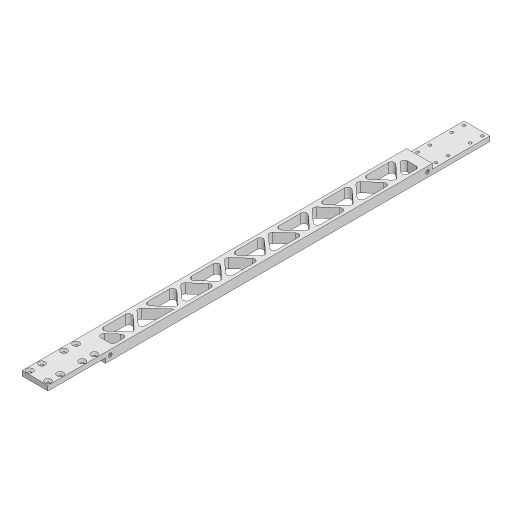
# Autodesk Inventor part: mgn7 300mm Connector Plate
Saved by Autodesk Inventor 2023 (Build 270158000, 158)
## iProperties
Created: 2022-09-25
Part Number: mgn7 300mm Connector Plate
Material: Generic
Document SubType Name: Modeling
Designer: deli
Density: 1 g/cm^3
Appearance: Default
Mass: 15.4529 g
Surface Area: 147.421 cm^2
Volume: 15.4529 cm^3
Author: deli
Autodesk Inventor part; units mm, degrees
ref_plane "YZ Plane" through (0, 0, 0) normal (1, 0, 0) x (0, 1, 0)
ref_plane "XZ Plane" through (0, 0, 0) normal (0, 1, 0) x (-1, 0, 0)
ref_plane "XY Plane" through (0, 0, 0) normal (0, 0, 1) x (1, 0, 0)
sketch "Sketch1" plane through (0, 0, 0) normal (0, 1, 0) x (-1, 0, 0)
  line L0 (25.6456, 320.9178) -> (8.6456, 320.9178)
  line L1 (8.6456, 320.9178) -> (8.6456, 30.4178)
  line L2 (8.6456, 30.4178) -> (25.6456, 30.4178)
  line L3 (25.6456, 30.4178) -> (25.6456, 320.9178)
  circle A0 centre (23.1456, 318.4178) radius 1
  circle A1 centre (23.1456, 310.4178) radius 1
  circle A2 centre (11.1456, 318.4178) radius 1
  circle A3 centre (11.1456, 310.4178) radius 1
  line L4 (23.1456, 318.4178) -> (23.1456, 310.4178) construction
  line L5 (23.1456, 310.4178) -> (11.1456, 310.4178) construction
  line L6 (11.1456, 310.4178) -> (11.1456, 318.4178) construction
  line L7 (11.1456, 318.4178) -> (23.1456, 318.4178) construction
  circle A4 centre (23.1456, 295.9178) radius 1
  circle A5 centre (23.1456, 287.9178) radius 1
  circle A6 centre (11.1456, 295.9178) radius 1
  circle A7 centre (11.1456, 287.9178) radius 1
  line L8 (23.1456, 295.9178) -> (23.1456, 287.9178) construction
  line L9 (23.1456, 287.9178) -> (11.1456, 287.9178) construction
  line L10 (11.1456, 287.9178) -> (11.1456, 295.9178) construction
  line L11 (11.1456, 295.9178) -> (23.1456, 295.9178) construction
  circle A8 centre (23.1456, 63.4178) radius 1
  circle A9 centre (23.1456, 55.4178) radius 1
  circle A10 centre (11.1456, 63.4178) radius 1
  circle A11 centre (11.1456, 55.4178) radius 1
  line L12 (23.1456, 63.4178) -> (23.1456, 55.4178) construction
  line L13 (23.1456, 55.4178) -> (11.1456, 55.4178) construction
  line L14 (11.1456, 55.4178) -> (11.1456, 63.4178) construction
  line L15 (11.1456, 63.4178) -> (23.1456, 63.4178) construction
  circle A12 centre (23.1456, 40.9178) radius 1
  circle A13 centre (23.1456, 32.9178) radius 1
  circle A14 centre (11.1456, 40.9178) radius 1
  circle A15 centre (11.1456, 32.9178) radius 1
  line L16 (23.1456, 40.9178) -> (23.1456, 32.9178) construction
  line L17 (23.1456, 32.9178) -> (11.1456, 32.9178) construction
  line L18 (11.1456, 32.9178) -> (11.1456, 40.9178) construction
  line L19 (11.1456, 40.9178) -> (23.1456, 40.9178) construction
  point P0 (0, 0)
  point P1 (17.1456, 30.4178)
  dimension "d0" = 17
  dimension "d23" = 2
  dimension "d24" = 2
  dimension "d25" = 2
  dimension "d26" = 2
  dimension "d27" = 12
  dimension "d28" = 8
  dimension "d29" = 2.5
  dimension "d31" = 2
  dimension "d32" = 2
  dimension "d33" = 2
  dimension "d34" = 2
  dimension "d35" = 8
  dimension "d36" = 12
  dimension "d38" = 14.5
  dimension "d49" = 8
  dimension "d50" = 12
  dimension "d58" = 8
  dimension "d59" = 12
  dimension "d63" = 14.5
  dimension "d94" = 224.5
  dimension "d101" = 285.5
  dimension "d107" = 2.5
  dimension "d108" = 2.5
  dimension "d213" = 2.5
  dimension "d214" = 2.5
  dimension "d215" = 2.5
  constraints: 40 end point, 16 centre point, 12 perpendicular, 8 equal radius, 4 vertical, 3 horizontal, 3 parallel, 1 midpoint
  measures "d0" distance of L2.end L1.end
  measures "d23" diameter of A0
  measures "d24" diameter of A1
  measures "d25" diameter of A2
  measures "d26" diameter of A3
  measures "d27" distance of L6.end L4.start
  measures "d28" distance of L4.start L4.end
  measures "d29" distance from line of L1 L6.end
  measures "d31" diameter of A4
  measures "d32" diameter of A5
  measures "d33" diameter of A6
  measures "d34" diameter of A7
  measures "d35" distance of L8.start L8.end
  measures "d36" distance of L10.end L8.start
  measures "d38" distance of L10.end L5.end
  measures "d49" distance of L12.end L15.end
  measures "d50" distance of L15.start L15.end
  measures "d58" distance of L19.end L16.end
  measures "d59" distance of L19.start L19.end
  measures "d63" distance of L14.start L19.start
  measures "d94" distance between parallel lines of L15 L9
  measures "d101" distance of L18.start L6.end
  measures "d107" distance from line of point (17.146, 30.418) L17
  measures "d108" distance between parallel lines of L0 L7
  measures "d213" distance between parallel lines of L1 L18
  measures "d214" distance between parallel lines of L1 L14
  measures "d215" distance between parallel lines of L1 L10
extrude "Extrusion1" add sketch "Sketch1" along normal blind 6.35
sketch "Sketch2" plane through (0, 6.35, 0) normal (0, 1, 0) x (1, 0, 0)
  line L0 (-8.6456, -30.4178) -> (-25.6456, -30.4178) projected
  line L1 (-8.6456, -320.9178) -> (-8.6456, -30.4178) projected
  line L2 (-25.6456, -30.4178) -> (-8.6456, -30.4178)
  line L3 (-8.6456, -30.4178) -> (-8.6456, -68.1678)
  line L4 (-8.6456, -68.1678) -> (-25.6456, -68.1678)
  line L5 (-25.6456, -68.1678) -> (-25.6456, -30.4178)
  point P0 (0, 0)
  dimension "d182" = 37.75
  constraints: 8 end point, 2 parallel, 1 horizontal, 1 perpendicular, 1 point on line
  measures "d182" distance of L2.end L3.end
extrude "Extrusion2" cut sketch "Sketch2" against normal blind 3.175
sketch "Sketch3" plane through (0, 0, 0) normal (0, -1, 0) x (1, 0, 0)
  line L0 (-25.6456, 30.4178) -> (-25.6456, 320.9178) projected
  line L1 (-8.6456, 320.9178) -> (-8.6456, 30.4178) projected
  line L2 (-25.6456, 320.9178) -> (-8.6456, 320.9178)
  line L3 (-8.6456, 320.9178) -> (-8.6456, 283.1678)
  line L4 (-8.6456, 283.1678) -> (-25.6456, 283.1678)
  line L5 (-25.6456, 283.1678) -> (-25.6456, 320.9178)
  point P0 (0, 0)
  point P1 (-8.6456, 320.9178)
  point P2 (-25.6456, 283.1678)
  dimension "d192" = 37.75
  constraints: 8 end point, 2 parallel, 1 horizontal, 1 perpendicular, 1 point on line
  measures "d192" distance of L2.end L3.end
extrude "Extrusion3" cut sketch "Sketch3" against normal blind 3.175
sketch "Sketch4" plane through (-8.6456, 6.35, 320.9178) normal (1, 0, 0) x (0, 0, -1)
  circle A0 centre (249.5, -3.175) radius 1.25
  line L0 (37.75, -6.35) -> (290.5, -6.35) projected
  line L1 (252.75, -3.175) -> (252.75, 0) projected
  circle A1 centre (41, -3.175) radius 1.25
  line L2 (37.75, -3.175) -> (37.75, -6.35) projected
  point P0 (320.9178, -6.35)
  dimension "d196" = 2.5
  dimension "d199" = 2
  dimension "d200" = 3.175
  dimension "d207" = 2.5
  dimension "d208" = 2
  dimension "d209" = 3.175
  constraints: 2 centre point
  measures "d196" diameter of A0
  measures "d199" distance edge to line of A0 L1
  measures "d200" distance from line of L0 A0.centre
  measures "d207" diameter of A1
  measures "d208" distance edge to line of A1 L2
  measures "d209" distance from line of A1.centre L0
extrude "Extrusion4" cut sketch "Sketch4" against normal blind 8
thread "Thread1" size "M3x0.5" class "6H" standard "ANSI Metric M Profile" full length
thread "Thread3" size "M3x0.5" class "6H" standard "ANSI Metric M Profile" full length
sketch "Sketch5" plane through (0, 6.35, 0) normal (0, 1, 0) x (1, 0, 0)
  line L0 (-8.6456, -68.1678) -> (-25.6456, -68.1678) projected
  line L1 (-8.6456, -283.1678) -> (-25.6456, -283.1678) projected
  line L2 (-25.6456, -283.1678) -> (-25.6456, -68.1678)
  line L3 (-8.6456, -68.1678) -> (-8.6456, -283.1678)
  line L4 (-23.6456, -77.5834) -> (-23.6456, -100.9939)
  line L5 (-23.6456, -100.9939) -> (-10.6456, -89.2887)
  line L6 (-10.6456, -89.2887) -> (-23.6456, -77.5834)
  line L7 (-23.6456, -74.8921) -> (-10.6456, -74.8921)
  line L8 (-10.6456, -74.8921) -> (-10.6456, -86.5974)
  line L9 (-10.6456, -86.5974) -> (-23.6456, -74.8921)
  line L10 (-10.6456, -91.9799) -> (-23.6456, -103.6852)
  line L11 (-23.6456, -103.6852) -> (-10.6456, -115.3904)
  line L12 (-10.6456, -115.3904) -> (-10.6456, -91.9799)
  line L13 (-23.6456, -106.3764) -> (-10.6456, -118.0817)
  line L14 (-10.6456, -118.0817) -> (-23.6456, -129.7869)
  line L15 (-23.6456, -129.7869) -> (-23.6456, -106.3764)
  line L16 (-10.6456, -120.773) -> (-23.6456, -132.4782)
  line L17 (-23.6456, -132.4782) -> (-10.6456, -144.1835)
  line L18 (-10.6456, -144.1835) -> (-10.6456, -120.773)
  line L19 (-23.6456, -135.1695) -> (-10.6456, -146.8747)
  line L20 (-10.6456, -146.8747) -> (-23.6456, -158.58)
  line L21 (-23.6456, -158.58) -> (-23.6456, -135.1695)
  line L22 (-10.6456, -149.566) -> (-23.6456, -161.2712)
  line L23 (-23.6456, -161.2712) -> (-10.6456, -172.9765)
  line L24 (-10.6456, -172.9765) -> (-10.6456, -149.566)
  line L25 (-23.6456, -163.9625) -> (-23.6456, -187.373)
  line L26 (-23.6456, -187.373) -> (-10.6456, -175.6678)
  line L27 (-10.6456, -175.6678) -> (-23.6456, -163.9625)
  line L28 (-10.6456, -178.359) -> (-23.6456, -190.0643)
  line L29 (-23.6456, -190.0643) -> (-10.6456, -201.7695)
  line L30 (-10.6456, -201.7695) -> (-10.6456, -178.359)
  line L31 (-23.6456, -192.7555) -> (-10.6456, -204.4608)
  line L32 (-10.6456, -204.4608) -> (-23.6456, -216.1661)
  line L33 (-23.6456, -216.1661) -> (-23.6456, -192.7555)
  line L34 (-23.6456, -276.4434) -> (-10.6456, -264.7381)
  line L35 (-23.6456, -276.4434) -> (-10.6456, -276.4434)
  line L36 (-10.6456, -264.7381) -> (-10.6456, -276.4434)
  line L37 (-7.6456, -67.1678) -> (-7.6456, -282.1678)
  line L38 (-10.6456, -207.1521) -> (-23.6456, -218.8573)
  line L39 (-23.6456, -218.8573) -> (-10.6456, -230.5626)
  line L40 (-10.6456, -230.5626) -> (-10.6456, -207.1521)
  line L41 (-23.6456, -221.5486) -> (-10.6456, -233.2538)
  line L42 (-10.6456, -233.2538) -> (-23.6456, -244.9591)
  line L43 (-23.6456, -244.9591) -> (-23.6456, -221.5486)
  line L44 (-6.6456, -66.1678) -> (-6.6456, -281.1678)
  line L45 (-10.6456, -235.9451) -> (-23.6456, -247.6504)
  line L46 (-23.6456, -247.6504) -> (-10.6456, -259.3556)
  line L47 (-10.6456, -259.3556) -> (-10.6456, -235.9451)
  line L48 (-23.6456, -250.3416) -> (-10.6456, -262.0469)
  line L49 (-10.6456, -262.0469) -> (-23.6456, -273.7521)
  line L50 (-23.6456, -273.7521) -> (-23.6456, -250.3416)
  point P0 (0, 0)
  point P1 (-10.6456, -188.3577)
  point P2 (-10.6456, -154.3183)
  point P3 (-23.6456, -306.5944)
  dimension "d216" = 48
  dimension "d217" = 2
  dimension "d218" = 2
  dimension "d219" = 6.7244
  dimension "d221" = 2
  dimension "d227" = 2
  dimension "d228" = 2
  dimension "d232" = 2
  dimension "d233" = 2
  dimension "d234" = 215
  dimension "d235" = 2
  dimension "d236" = 2
  dimension "d237" = 2
  dimension "d238" = 2
  dimension "d240" = 201.5513
  dimension "d244" = 2
  dimension "d252" = 2
  dimension "d253" = 2
  dimension "d261" = 2
  dimension "d262" = 2
  constraints: 98 end point, 27 parallel, 22 point on line, 15 equal length, 6 collinear, 3 perpendicular, 3 vertical, 1 horizontal
  measures "d216" angle of L6 L4
  measures "d217" distance between parallel lines of L2 L4
  measures "d218" distance between parallel lines of L3 L8
  measures "d219" distance between parallel lines of L0 L7
  measures "d221" distance from line of L6 L7.start
  measures "d227" distance between parallel lines of L10 L5
  measures "d228" distance between parallel lines of L11 L13
  measures "d232" distance between parallel lines of L16 L14
  measures "d233" distance between parallel lines of L17 L19
  measures "d234" distance between parallel lines of L1 L0
  measures "d235" distance between parallel lines of L22 L20
  measures "d236" distance between parallel lines of L23 L27
  measures "d237" distance between parallel lines of L28 L26
  measures "d238" distance between parallel lines of L29 L31
  measures "d240" distance between parallel lines of L7 L35
  measures "d244" distance between parallel lines of L39 L41
  measures "d252" distance between parallel lines of L38 L32
  measures "d253" distance between parallel lines of L46 L48
  measures "d261" distance between parallel lines of L34 L49
  measures "d262" distance between parallel lines of L42 L45
extrude "Extrusion5" cut sketch "Sketch5" against normal blind 10 contours L6 L5 L4 | L7 L8 L9 | L12 L11 L10 | L13 L14 L15 | L18 L17 L16 | L19 L20 L21 | L24 L23 L22 | L27 L26 L25 | L30 L29 L28 | L31 L32 L33 | L34 L36 L35 | L40 L39 L38 | L41 L42 L43 | L47 L46 L45 | L48 L49 L50
fillet "Fillet3" radius 2 44 edges at (-10.6456, 3.175, 276.4434) (-23.6456, 3.175, 276.4434) (-10.6456, 3.175, 264.7381) (-23.6456, 3.175, 216.1661) (-10.6456, 3.175, 204.4608) (-23.6456, 3.175, 192.7555) (-23.6456, 3.175, 190.0643) (-10.6456, 3.175, 201.7695) (-10.6456, 3.175, 178.359) (-23.6456, 3.175, 187.373) (-10.6456, 3.175, 175.6678) (-23.6456, 3.175, 163.9625) (-23.6456, 3.175, 161.2712) (-10.6456, 3.175, 172.9765) (-10.6456, 3.175, 149.566) (-23.6456, 3.175, 158.58) (-10.6456, 3.175, 146.8747) (-23.6456, 3.175, 135.1695) (-23.6456, 3.175, 132.4782) (-23.6456, 3.175, 129.7869) (-10.6456, 3.175, 144.1835) (-10.6456, 3.175, 120.773) (-10.6456, 3.175, 118.0817) (-10.6456, 3.175, 115.3904) (-23.6456, 3.175, 106.3764) (-23.6456, 3.175, 103.6852) (-23.6456, 3.175, 100.9939) (-10.6456, 3.175, 91.9799) (-10.6456, 3.175, 89.2887) (-10.6456, 3.175, 86.5974) (-23.6456, 3.175, 77.5834) (-23.6456, 3.175, 74.8921) (-10.6456, 3.175, 74.8921) (-10.6456, 3.175, 207.1521) (-23.6456, 3.175, 218.8573) (-10.6456, 3.175, 230.5626) (-10.6456, 3.175, 233.2538) (-23.6456, 3.175, 221.5486) (-23.6456, 3.175, 247.6504) (-23.6456, 3.175, 244.9591) (-23.6456, 3.175, 250.3416) (-10.6456, 3.175, 259.3556) (-10.6456, 3.175, 262.0469) (-23.6456, 3.175, 273.7521)
chamfer "Chamfer1" distance 1.2 angle 45 16 edges at (-10.1456, 6.35, 318.4178) (-22.1456, 6.35, 318.4178) (-22.1456, 6.35, 310.4178) (-10.1456, 6.35, 310.4178) (-22.1456, 6.35, 295.9178) (-10.1456, 6.35, 295.9178) (-22.1456, 6.35, 287.9178) (-10.1456, 6.35, 287.9178) (-22.1456, 0, 63.4178) (-10.1456, 0, 55.4178) (-10.1456, 0, 63.4178) (-10.1456, 0, 40.9178) (-10.1456, 0, 32.9178) (-22.1456, 0, 32.9178) (-22.1456, 0, 40.9178) (-22.1456, 0, 55.4178)
equation "\"d24\" = d23"
equation "\"d25\" = d23"
equation "\"d26\" = d23"
equation "\"d29\" = -0.5 * d27 + 0.5 * d0"
equation "\"d31\" = d23"
equation "\"d32\" = d23"
equation "\"d33\" = d23"
equation "\"d34\" = d23"
equation "\"d35\" = d28"
equation "\"d36\" = d27"
equation "\"d63\" = d38"
body "Solid1"
